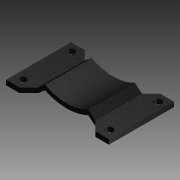
# Autodesk Inventor part: mount plate
Saved by Autodesk Inventor 2012 (Build 160160000, 160)
## iProperties
Created: 2012-02-04
Part Number: mount plate
Material: Steel
Document SubType Name: Modeling
Designer: Antonella Wilby
Density: 7.85 g/cm^3
Mass: 305.461 g
Surface Area: 169.801 cm^2
Volume: 38.9123 cm^3
Author: Antonella Wilby
Autodesk Inventor part; units mm, degrees
ref_plane "YZ Plane" through (0, 0, 0) normal (1, 0, 0) x (0, 1, 0)
ref_plane "XZ Plane" through (0, 0, 0) normal (0, 1, 0) x (-1, 0, 0)
ref_plane "XY Plane" through (0, 0, 0) normal (0, 0, 1) x (1, 0, 0)
sketch "Sketch1" plane through (0, 0, 0) normal (0, 0, 1) x (1, 0, 0)
  line L0 (-84.455, 0) -> (84.455, 0) projected
  line L1 (0, -53.34) -> (0, 53.34) projected
  line L2 (60.325, 38.1) -> (60.325, -38.1)
  line L3 (-60.325, -38.1) -> (-60.325, 38.1)
  line L4 (44.45, 38.1) -> (44.45, -38.1) construction
  line L5 (-44.45, -38.1) -> (-44.45, 38.1) construction
  line L6 (-33.655, -27.305) -> (33.655, -27.305)
  line L7 (-44.45, 38.1) -> (-33.655, 27.305)
  line L8 (-60.325, 38.1) -> (-44.45, 38.1)
  line L9 (44.45, 38.1) -> (60.325, 38.1)
  line L10 (33.655, 27.305) -> (-33.655, 27.305)
  line L11 (33.655, 27.305) -> (44.45, 38.1)
  line L12 (-44.45, -38.1) -> (-33.655, -27.305)
  line L13 (44.45, -38.1) -> (33.655, -27.305)
  line L14 (60.325, -38.1) -> (44.45, -38.1)
  line L15 (-44.45, -38.1) -> (-60.325, -38.1)
  point P0 (0, 0)
  point P1 (-60.325, 0)
  point P2 (0, 27.305)
  dimension "d1" = 76.2
  dimension "d2" = 15.875
  dimension "d4" = 45
  dimension "d5" = 54.61
  dimension "d6" = 120.65
  dimension "d7" = 15.875
  dimension "d8" = 45
  dimension "d9" = 10.795
  constraints: 28 end point, 9 parallel, 3 perpendicular, 2 collinear, 2 horizontal, 2 midpoint, 1 horizontal alignment, 1 vertical alignment
  measures "d1" distance of L3.start L3.end
  measures "d2" distance between parallel lines of L3 L5
  measures "d4" angle of L7 L5
  measures "d5" distance between parallel lines of L10 L6
  measures "d6" distance between parallel lines of L2 L3
  measures "d7" distance between parallel lines of L2 L4
  measures "d8" angle of L4 L11
  measures "d9" distance between parallel lines of L8 L10
extrude "Extrusion1" add sketch "Sketch1" against normal blind 12.7
sketch "Sketch2" plane through (-33.655, 27.305, 0) normal (0, 1, 0) x (1, 0, 0)
  line L0 (67.31, 12.7) -> (0, 12.7) projected
  line L1 (67.31, 0) -> (67.31, 12.7) projected
  line L2 (0, 12.7) -> (-10.795, 12.7) projected
  line L3 (-10.795, 0) -> (-10.795, 12.7) projected
  line L4 (0, 0) -> (-10.795, 0) projected
  line L5 (0, 0) -> (0, 12.7) projected
  line L6 (-10.795, 12.7) -> (-26.67, 12.7) projected
  line L7 (-26.67, 0) -> (-26.67, 12.7) projected
  line L8 (-10.795, 0) -> (-26.67, 0) projected
  line L9 (-10.795, 0) -> (-10.795, 12.7) projected
  line L10 (-10.795, 12.7) -> (-26.67, 12.7) projected
  line L11 (-26.67, 0) -> (-26.67, 12.7) projected
  line L12 (-10.795, 0) -> (-10.795, 12.7) projected
  line L13 (93.98, 0) -> (78.105, 0) projected
  line L14 (78.105, 0) -> (67.31, 0) projected
  line L15 (78.105, 0) -> (78.105, 12.7) projected
  line L16 (78.105, 12.7) -> (67.31, 12.7) projected
  line L17 (93.98, 12.7) -> (78.105, 12.7) projected
  line L18 (93.98, 12.7) -> (78.105, 12.7) projected
  line L19 (78.105, 0) -> (78.105, 12.7) projected
  line L20 (93.98, 0) -> (78.105, 0) projected
  line L21 (93.98, 0) -> (93.98, 12.7) projected
  line L22 (33.655, 0) -> (33.655, 12.7) construction
  line L23 (59.055, 0) -> (59.055, 12.7) construction
  line L24 (8.255, 0.2933) -> (8.255, 12.9933) construction
  arc A0 (8.255, 7.0115) -> (59.055, 7.0115) centre (33.655, 60.325) ccw
  arc A1 (8.255, 12.7) -> (59.055, 12.7) centre (33.655, 60.325) ccw
  line L25 (66.421, 0.7551) -> (59.055, 7.0115)
  line L26 (59.055, 12.7) -> (67.31, 5.6885)
  line L27 (68.4764, 0) -> (93.98, 0)
  arc A2 (66.421, 0.7551) -> (68.4764, 0) centre (68.4764, 3.175) ccw
  line L28 (67.31, 5.6885) -> (93.98, 5.6885)
  line L29 (93.98, 0) -> (93.98, 5.6885)
  line L30 (0.889, 0.7551) -> (8.255, 7.0115)
  line L31 (8.255, 12.7) -> (0, 5.6885)
  line L32 (-1.1664, 0) -> (-26.67, 0)
  line L33 (0, 5.6885) -> (-26.67, 5.6885)
  line L34 (-26.67, 0) -> (-26.67, 5.6885)
  arc A3 (-1.1664, 0) -> (0.889, 0.7551) centre (-1.1664, 3.175) ccw
  dimension "d12" = 50.8
  dimension "d13" = 53.975
  dimension "d14" = 5.08
  dimension "d15" = 3.175
  dimension "d17" = 3.175
  constraints: 26 end point, 14 point on line, 9 point on circle, 5 parallel, 4 centre point, 4 collinear, 4 tangent, 1 horizontal alignment, 1 midpoint, 1 perpendicular, 1 other
  measures "d12" distance between parallel lines of L23 L24
  measures "d13" radius of A1
  measures "d14" radial gap between concentric circles of A1 A0
  measures "d15" radius of A2
  measures "d17" radius of A3
extrude "Extrusion2" cut sketch "Sketch2" along normal through all both and the other way through all contours L26 L1 A2 L25 A0 L30 A3 L5 L31 A1 | L28 L15 L14 A2 L1 | L28 L21 L13 L15 | L5 A3 L4 L3 L33 | L3 L8 L7 L33 keep common part
sketch "Sketch3" plane through (60.325, 38.1, -5.6885) normal (0, 0, -1) x (-1, 0, 0)
  line L0 (0, 0) -> (0, -76.2) projected
  line L1 (26.67, -65.405) -> (26.67, -10.795) projected
  line L2 (0, -38.1) -> (26.67, -38.1) construction
  point P0 (60.325, -38.1)
  point P1 (9.271, -9.525)
  point P2 (9.271, -66.675)
  dimension "d20" = 57.15
  dimension "d21" = 9.271
  constraints: 2 end point, 2 midpoint, 1 symmetric about line, 1 vertical alignment
  measures "d20" distance of point (9.271, -9.525) point (9.271, -66.675)
  measures "d21" distance from line of L0 point (9.271, -9.525)
hole "Hole1" at (51.054, 28.575, -5.6885) at (51.054, -28.575, -5.6885) direction (0, 0, 1) diameter 8.89 end through all
mirror "Mirror1" about plane through (0, 0, 0) normal (1, 0, 0) of "Hole1"
equation "\"d9\" = -0.5 * d5 + 0.5 * d1"
body "Solid1"
